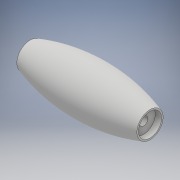
# Autodesk Inventor part: RollerRedesign5
Saved by Autodesk Inventor 2018 (Build 220112000, 112)
## iProperties
Created: 2017-08-15
Part Number: RollerRedesign5
Material: Generic
Document SubType Name: Modeling
Designer: P136265
Density: 1 g/cm^3
Appearance: Default
Mass: 135.616 g
Surface Area: 153.177 cm^2
Volume: 135.616 cm^3
Author: P136265
Autodesk Inventor part; units mm, degrees
ref_plane "YZ Plane" through (0, 0, 0) normal (1, 0, 0) x (0, 1, 0)
ref_plane "XZ Plane" through (0, 0, 0) normal (0, 1, 0) x (-1, 0, 0)
ref_plane "Work Plane1" through (0, 0, 0) normal (0, -0.7071068, 0.7071068) x (1, 0, 0)
sketch "Sketch1" plane through (0, 0, 0) normal (0, -0.7071068, 0.7071068) x (1, 0, 0)
  circle A0 centre (0, 0) radius 100 construction
  dimension "d1" = 200
  constraints: 1 centre point, 1 coincident
  measures "d1" diameter of A0
sketch "Sketch2" plane through (0, 0, 0) normal (0, 0, 1) x (1, 0, 0)
  line L0 (0, 0) -> (0, 100) construction
  line L1 (0, 0) -> (135.52, 0) construction
  circle A0 centre (0, 74.9294) radius 25 construction
  circle A1 centre (0, 74.9294) radius 12.5 construction
  line L2 (89.6381, 86.81) -> (-89.6381, 86.81) construction
  line L3 (-67.2707, 86.81) -> (-67.2707, 75) construction
  line L4 (-65.5817, 87.4347) -> (-65.5817, 74.9294) construction
  line L5 (65.5817, 87.4347) -> (65.5817, 74.9294) construction
  ellipse E0 centre (0, 0) end of major axis (135.4472, 0) minor radius 99.9294 (65.5817, 87.4347) -> (-65.5817, 87.4347) ccw construction
  line L6 (-62.6083, 85.4701) -> (-62.6083, 74.9294) construction
  line L7 (62.5858, 74.9294) -> (62.5858, 85.4128) construction
  line L8 (-57.1593, 87.4294) -> (-57.1593, 74.9294)
  line L9 (57.1593, 87.4294) -> (-57.1593, 87.4294) construction
  line L10 (57.1593, 87.4294) -> (57.1593, 74.9294)
  line L11 (57.1593, 74.9294) -> (-57.1593, 74.9294)
  spline S0 degree 5 poles (57.1593, 87.4294) (46.1717, 91.2827) (34.8288, 94.1238) (23.2875, 95.9996) (0, 97.8773) (-23.2875, 95.9996) (-34.8288, 94.1238) (-46.1717, 91.2827) (-57.1593, 87.4294) knots 0 0 0 0 0 0 0.5 0.5 0.5 1 1 1 1 1 1
  dimension "d40" = 135.4471
  dimension "d41" = 99.9294
  dimension "d24" = 50
  dimension "d25" = 0
  dimension "d26" = 25
  dimension "d42" = 86.81
  dimension "d43" = 2.9958
  dimension "d44" = 8.4224
  dimension "d45" = 65.5817
  dimension "d46" = 128.19
  dimension "d47" = 132.8524
  dimension "d48" = 0
  dimension "d49" = 65.5817
  dimension "d50" = 69.9383
  dimension "d51" = 24.0564
  dimension "d52" = 74.9294
  dimension "d53" = 85.4129
  dimension "d54" = 74.9294
  dimension "d55" = 100
  dimension "d56" = 85.4701
  dimension "d57" = 74.9294
  dimension "d58" = 75
  dimension "d59" = 155.2197
  constraints: 24 end point, 4 parallel, 4 perpendicular, 3 horizontal, 2 centre point, 2 coincident, 2 symmetric about line, 1 horizontal alignment, 1 midpoint, 1 point on line, 1 tangent, 1 vertical, 7 other
  measures "d24" diameter of A0
  measures "d25" horizontal distance of L0.start A0.centre
  measures "d26" diameter of A1
  measures "d42" distance between parallel lines of L1 L2
  measures "d43" distance between parallel lines of L5 L7
  measures "d44" distance between parallel lines of L5 L10
  measures "d45" distance between parallel lines of L5 L0
  measures "d46" distance between parallel lines of L5 L6
  measures "d47" distance between parallel lines of L5 L3
  measures "d48" distance from line of point (0, 0) L1
  measures "d49" distance from line of point (0, 0) L5
  measures "d50" distance from line of L1.end L5
  measures "d51" distance from line of L2.start L5
  measures "d52" distance from line of L5.end L1
  measures "d53" distance from line of L7.end L1
  measures "d54" distance from line of L7.start L1
  measures "d55" distance from line of L0.end L1
  measures "d56" distance from line of L6.start L1
  measures "d57" distance from line of L6.end L1
  measures "d58" distance from line of L3.end L1
  measures "d59" distance from line of L2.end L5
revolve "Revolution3" add sketch "Sketch2" angle 360 about axis through (57.1593, 74.9294, 0) along (-1, 0, 0)
sketch "Sketch6" plane through (-57.1593, 74.9294, 0) normal (-1, 0, 0) x (0, 0, 1)
  circle A0 centre (0, 0) radius 12.5 projected
  circle A1 centre (0, 0) radius 11
  point P0 (0, -74.9294)
  point P1 (0, 12.5)
  dimension "d61" = 22
  constraints: 1 centre point, 1 coincident, 1 vertical alignment
  measures "d61" diameter of A1
extrude "Extrusion3" cut sketch "Sketch6" against normal blind 6 contours A1
sketch "Sketch7" plane through (57.1593, 74.9294, 0) normal (1, 0, 0) x (0, 0, -1)
  circle A0 centre (0, 0) radius 12.5 projected
  circle A1 centre (0, 0) radius 11
  point P0 (0, -74.9294)
  point P1 (0, 12.5)
  dimension "d64" = 22
  constraints: 1 centre point, 1 coincident, 1 vertical alignment
  measures "d64" diameter of A1
extrude "Extrusion4" cut sketch "Sketch7" against normal blind 6 contours A1
hole "Hole2" at (57.1593, 74.9294, 0) direction (-1, 0, 0) diameter 8 end through all
body "Solid3"
